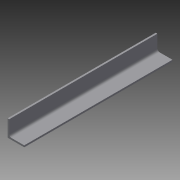
# Autodesk Inventor part: hubRingJigOuter
Saved by Autodesk Inventor 2014 (Build 180170000, 170)
## iProperties
Created: 2014-12-02
Part Number: hubRingJigOuter
Material: Generic
Document SubType Name: Modeling
Designer: Dave
Density: 1 g/cm^3
Appearance: Default
Author: Dave
Autodesk Inventor part; units mm, degrees
ref_plane "YZ Plane" through (0, 0, 0) normal (1, 0, 0) x (0, 1, 0)
ref_plane "XZ Plane" through (0, 0, 0) normal (0, 1, 0) x (-1, 0, 0)
ref_plane "XY Plane" through (0, 0, 0) normal (0, 0, 1) x (1, 0, 0)
sketch "Sketch1" plane through (0, 0, 0) normal (0, 0, 1) x (1, 0, 0)
  line L0 (0, 0) -> (0, 25.4)
  line L1 (0, 0) -> (25.4, 0)
  line L2 (2.54, 25.4) -> (2.54, 5.715)
  line L3 (5.715, 2.54) -> (25.4, 2.54)
  arc A0 (2.54, 5.715) -> (5.715, 2.54) centre (5.715, 5.715) ccw
  line L4 (0, 25.4) -> (2.54, 25.4)
  line L5 (25.4, 2.54) -> (25.4, 0)
  dimension "d0" = 25.4
  dimension "d1" = 25.4
  dimension "d2" = 2.54
  dimension "d3" = 3.175
  constraints: 12 end point, 3 perpendicular, 2 point on circle, 2 tangent, 1 centre point, 1 parallel, 1 vertical, 1 other
  measures "d0" distance of L0.start L0.end
  measures "d1" distance of L0.start L1.end
  measures "d2" distance between parallel lines of L2 L0
  measures "d3" radius of A0
extrude "Extrusion1" add sketch "Sketch1" along normal blind 225
sketch "Sketch4" plane through (0, 0, 0) normal (-1, 0, 0) x (0, 0, 1)
  line L0 (0, 0) -> (0, 25.4) projected
  line L1 (0, 0) -> (225, 0) projected
  line L2 (0, 25.4) -> (225, 25.4) projected
  line L3 (38.1, 6.985) -> (88.9, 6.985) construction
  line L4 (38.1, 3.81) -> (88.9, 3.81)
  line L5 (88.9, 10.16) -> (38.1, 10.16)
  arc A0 (38.1, 10.16) -> (38.1, 3.81) centre (38.1, 6.985) ccw
  arc A1 (88.9, 3.81) -> (88.9, 10.16) centre (88.9, 6.985) ccw
  line L6 (112.5, 25.4) -> (112.5, 0) construction
  point P0 (63.5, 6.985)
  dimension "d19" = 50.8
  dimension "d20" = 6.35
  dimension "d21" = 3.81
  dimension "d22" = 63.5
  constraints: 10 end point, 4 point on circle, 4 tangent, 3 midpoint, 2 centre point, 2 parallel
  measures "d19" distance of L3.start L3.end
  measures "d20" diameter of A1
  measures "d21" distance between parallel lines of L1 L4
  measures "d22" distance from line of point (63.5, 6.985) L0
extrude "Extrusion4" [suppressed]
sketch "Sketch5" plane through (0, 0, 0) normal (0, -1, 0) x (1, 0, 0)
  line L0 (25.4, 0) -> (0, 0) projected
  line L1 (25.4, 0) -> (25.4, 225) projected
  line L2 (0, 0) -> (0, 225) projected
  line L3 (0, 182.555) -> (25.4, 182.555)
  constraints: 2 end point, 2 point on line, 1 perpendicular
extrude "Extrusion5" [suppressed]
equation "\"d27\" = 0.5 * hubAngleThickness"
equation "\"hubAngleThickness\" = 3"
equation "\"hubAngleWidth1\" = 25.4"
equation "\"hubAngleWidth2\" = 25.4"
body "Solid1"
